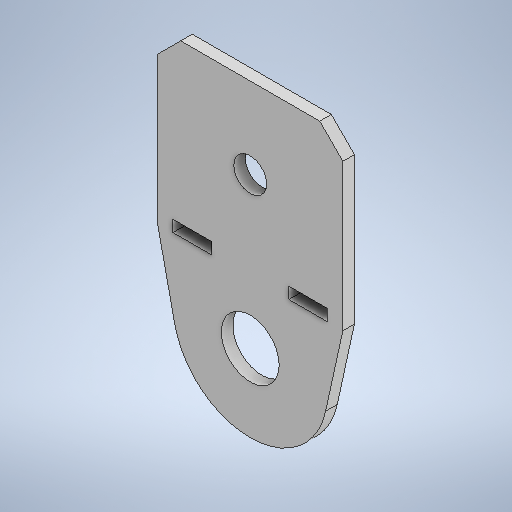
# Autodesk Inventor part: A_beam_end_mound_2
Saved by Autodesk Inventor 2025.2 (Build 292293000, 293)
## iProperties
Created: 2025-05-02
Part Number: A_beam_end_mound_2
Material: Generic
Document SubType Name: Sheet Metal
Designer: Caspe
Density: 1 g/cm^3
Sheet Metal Rule: Default_mm
Appearance: Default
Author: Caspe
Autodesk Inventor part; units mm, degrees
ref_plane "YZ Plane" through (0, 0, 0) normal (1, 0, 0) x (0, 1, 0)
ref_plane "XZ Plane" through (0, 0, 0) normal (0, 1, 0) x (-1, 0, 0)
ref_plane "XY Plane" through (0, 0, 0) normal (0, 0, 1) x (1, 0, 0)
sketch "Sketch1" plane through (0, 0, 0) normal (0, 0, 1) x (1, 0, 0)
  line L0 (0, 0) -> (10, 0)
  line L1 (10, 0) -> (10, 3)
  line L2 (10, 3) -> (0, 3)
  line L3 (0, 3) -> (0, 0)
  line L4 (30, 0) -> (40, 0)
  line L5 (40, 0) -> (40, 3)
  line L6 (40, 3) -> (30, 3)
  line L7 (30, 3) -> (30, 0)
  line L8 (0, 0) -> (40, 0)
  line L9 (40, 0) -> (40, 40)
  line L10 (40, 40) -> (0, 40)
  line L11 (0, 40) -> (0, 0)
  circle A0 centre (20, -16) radius 7.5
  circle A1 centre (20, -16) radius 20
  line L12 (-4, 44) -> (44, 44)
  line L13 (44, 44) -> (44, 0)
  line L14 (44, 0) -> (-4, 0)
  line L15 (-4, 0) -> (-4, 44)
  line L16 (-4, 0) -> (0.4675, -20.2988)
  line L17 (44, 0) -> (39.5325, -20.2988)
  circle A2 centre (20, 23) radius 4.25
  line L18 (10, 3) -> (30, 3)
  point P0 (20, 0)
  point P1 (1.3083, -23.1147)
  point P2 (38.6917, -23.1147)
  point P3 (30, 1.3205)
  point P4 (10, 1.3205)
  point P5 (8, 0)
  point P6 (32, 0)
  dimension "d0" = 10
  dimension "d1" = 3
  dimension "d2" = 10
  dimension "d3" = 20
  dimension "d4" = 40
  dimension "d5" = 15
  dimension "d6" = 40
  dimension "d7" = 16
  dimension "d9" = 4
  dimension "d10" = 4
  dimension "d11" = 4
  dimension "d12" = 8.5
  dimension "d17" = 20
  measures "d0" distance of L2.end L1.end
  measures "d1" distance of L1.end L0.end
  measures "d2" distance of L6.end L5.end
  measures "d3" distance between parallel lines of L7 L1
  measures "d4" distance of L9.end L8.end
  measures "d5" diameter of A0
  measures "d6" diameter of A1
  measures "d7" distance of point (20, 0) A1.centre
  measures "d9" distance between parallel lines of L11 L15
  measures "d10" distance between parallel lines of L12 L10
  measures "d11" distance between parallel lines of L13 L9
  measures "d12" diameter of A2
  measures "d17" distance from line of A2.centre L18
extrude "Plate1" add sketch "Sketch1" along normal blind 3 contours L14 L15 L12 L13 L5 L9 L10 L11 L3 | L0 A1 L16 L14 | L0 L8 L4 A1 | L11 L10 L9 L6 L18 A1 L2 | L1 A1 L18 L7 L8 | L1 L18 A1 | A1 L18 | A1 L4 L14 L17 | A1 L18 L7
chamfer "Corner Chamfer1" distance 6 angle 45 2 edges at (-4, 44, 1.5) (44, 44, 1.5)
equation "\"d10\" = d9"
equation "\"d11\" = d10"
equation "\"d8\" = Thickness"
equation "\"BendRadius\" = Thickness"
equation "\"BendReliefWidth\" = Thickness"
equation "\"BendReliefDepth\" = 0.5 * Thickness"
equation "\"CornerReliefSize\" = 4 * Thickness"
equation "\"MinimumRemnant\" = 2 * Thickness"
equation "\"TransitionRadius\" = BendRadius"
equation "\"JacobiRadiusSize\" = BendRadius"
equation "\"GapSize\" = Thickness"
equation "\"Thickness\" = 3"
body "Solid1"
